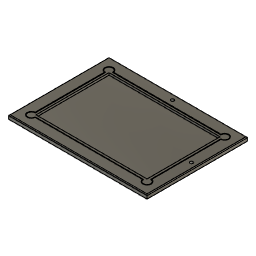
Honeycomb Frame (Autodesk Fusion 360 design; units mm, degrees)
Autodesk Fusion 360 part; units mm, degrees
note: some values were not read from the file. Set by a fixed rule: which face or edge a step refers to.
sketch "Skizze2" plane through (0, 0, 0) normal (0, 0, 1) x (1, 0, 0)
  line L0 (0, 0) -> (152, 0)
  line L1 (152, 0) -> (152, 102)
  line L2 (152, 102) -> (0, 102)
  line L3 (0, 102) -> (0, 0)
  line L4 (-15, 117) -> (-15, -15)
  line L5 (-15, -15) -> (167, -15)
  line L6 (167, -15) -> (167, 117)
  line L7 (167, 117) -> (-15, 117)
  line L8 (149, 3) -> (149, 99)
  line L9 (149, 99) -> (3, 99)
  line L10 (3, 99) -> (3, 3)
  line L11 (3, 3) -> (149, 3)
  circle A0 centre (76, 109.5) radius 2
  line L12 (76, 109.5) -> (76, 102) construction
  line L13 (76, 109.5) -> (76, 117) construction
  line L14 (76, 109.5) -> (-15, 109.5) construction
  line L15 (76, 109.5) -> (167, 109.5) construction
  line L16 (167, 117) -> (167, -15) construction
  line L17 (152, 102) -> (167, 102) construction
  line L18 (159.5, -77.2787) -> (159.5, -15) construction
  line L19 (152, 0) -> (167, 0) construction
  circle A1 centre (159.5, 51) radius 2
  line L20 (159.5, 117) -> (159.5, -15) construction
  line L21 (152, 51) -> (167, 51) construction
  dimension "d4" = 152
  dimension "d5" = 102
  dimension "d6" = 15
  dimension "d7" = -3
  dimension "d33" = 4
  dimension "d72" = 4
  constraint horizontal L0
  constraint vertical L1
  constraint horizontal L2
  constraint vertical L3
  constraint coincident L0.start L3.end
  constraint coincident A0.centre L12.start
  constraint coincident L2 L12.end
  constraint perpendicular L2 L12
  constraint coincident L7 L13.end
  constraint perpendicular L7 L13
  constraint equal L12 L13
  constraint coincident L4 L14.end
  constraint perpendicular L4 L14
  constraint coincident L6 L15.end
  constraint perpendicular L6 L15
  constraint equal L14 L15
  constraint coincident L7 L6.end
  constraint coincident L5 L6.start
  constraint perpendicular L5 L16
  constraint coincident L6 L17.end
  constraint perpendicular L6 L17
  constraint coincident L5 L18.end
  constraint perpendicular L5 L18
  constraint coincident L6 L19.end
  constraint perpendicular L6 L19
  constraint vertical L20
  constraint coincident L7 L20.start
  constraint coincident L1 L21.start
  constraint coincident L6 L21.end
  constraint perpendicular L6 L21
  constraint midpoint L20 L21
  constraint midpoint A1.centre L21
  measures "d4" distance of L0.start L0.end
  measures "d5" distance of L0.start L2.end
  measures "d33" diameter of A0
  measures "d72" diameter of A1
extrude "Extrusion1" add sketch "Skizze2" along normal blind 5 contours L4 L5 L6 L7 makes body 1
extrude "Extrusion2" add sketch "Skizze2" along normal blind 1 contours L0 L1 L2 L3 | L8 L9 L10 L11 bodies 1
sketch "Skizze6" plane through (0, 0, 5) normal (0, 0, 1) x (-1, 0, 0)
  circle A0 centre (-76, -109.5) radius 2
  line L0 (0, 0) -> (0, -102)
  line L1 (0, -102) -> (-152, -102)
  line L2 (-152, -102) -> (-152, 0)
  line L3 (-152, 0) -> (0, 0)
  line L4 (-167, -117) -> (15, -117)
  line L5 (15, -117) -> (15, 15)
  line L6 (15, 15) -> (-167, 15)
  line L7 (-167, 15) -> (-167, -117)
  line L8 (-3, -3) -> (-149, -3)
  line L9 (-149, -3) -> (-149, -99)
  line L10 (-149, -99) -> (-3, -99)
  line L11 (-3, -99) -> (-3, -3)
  line L12 (-152, 0) -> (-152, -102)
  line L13 (-152, -102) -> (0, -102)
  line L14 (0, -102) -> (0, 0)
  line L15 (0, 0) -> (-152, 0)
  circle A1 centre (0, -102) radius 5
  circle A2 centre (-152, 0) radius 5
  circle A3 centre (0, 0) radius 5
  circle A4 centre (-152, -102) radius 5
  circle A5 centre (-159.5, -51) radius 2
  dimension "d65" = 146
  dimension "d66" = 96
  dimension "d67" = 3
  dimension "d68" = 10
  dimension "d69" = 10
  dimension "d70" = 10
  dimension "d71" = 10
  constraint horizontal L8
  constraint vertical L9
  constraint horizontal L10
  constraint vertical L11
  constraint coincident L0.end L1.start
  constraint coincident L2.end L3.start
  constraint coincident L0.start L3.end
  constraint coincident L1.end L2.start
  measures "d65" distance of L8.start L8.end
  measures "d66" distance of L8.start L10.end
  measures "d68" diameter of A1
  measures "d69" diameter of A2
  measures "d70" diameter of A3
  measures "d71" diameter of A4
extrude "Extrusion7" add sketch "Skizze6" against normal blind 3 separate body contours L0 L3 L14 L15 A3 | L0 L3 L8 L11 L14 L15 A3 | L0 L11 L14 A1 A3 | L3 L8 L15 A2 A3 | L0 L1 L13 L14 A1 | L0 L1 L10 L11 L13 L14 A1 | L2 L3 L8 L9 L12 L15 A2 | L2 L3 L12 L15 A2 | L2 L9 L12 A2 A4 | L1 L10 L13 A1 A4 | L1 L2 L9 L10 L12 L13 A4 | L1 L2 L12 L13 A4 makes body 2
combine "Kombinieren2" operation cut target body 1 tool bodies 2 keep tools
move_face "Flächen versetzen4" offset -0.1 5 faces at (0, 35.6667, 3) (99.6667, 0, 3) (52.3333, 102, 3) (152, 66.3333, 4) (99.6667, 2, 2) on bodies 2
move_face "Flächen versetzen5" offset -0.1 6 faces at (152.1475, 4.9978, 3.0667) (155.8677, 105.1687, 4.0333) (-2.8755, -4.0904, 3.0667) (-4.4302, 2.318, 3.0667) (4.88, 103.0888, 3.0667) (-4.0499, 99.0677, 3.0667) on bodies 2
fillet "Abrundung5" radius 1 4 edges at (-15, 51, 5) (76, 117, 5) (76, -15, 5) (167, 51, 5) on bodies 1
fillet "Abrundung6" radius 0.5 8 edges at (-3.5355, 105.5355, 5) (76, 102, 5) (0, 51, 5) (-3.5355, -3.5355, 5) (76, 0, 5) (152, 51, 5) (155.5355, 105.5355, 5) (155.5355, -3.5355, 5) on bodies 1
equation "Fotobreite = 150 mm"
equation "Fotohöhe = 100 mm"
equation "d4 = Fotobreite + 2 mm"
equation "d5 = Fotohöhe + 2 mm"
equation "d65 = Fotobreite - 4 mm"
equation "d66 = Fotohöhe - 4 mm"
named bodies: "Frame_outer", "Frame_inner"
